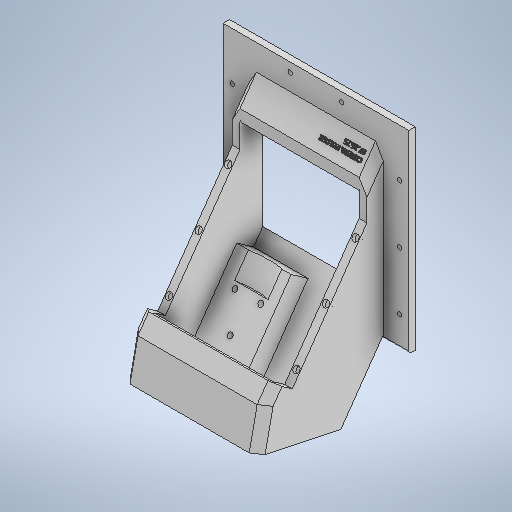
# Autodesk Inventor part: holderforcameras
Saved by Autodesk Inventor 2025.2 (Build 292293000, 293)
## iProperties
Created: 2025-07-10
Part Number: holderforcameras
Material: Generic
Document SubType Name: Modeling
Designer: mateo
Density: 1 g/cm^3
Appearance: Default
Author: mateo
Autodesk Inventor part; units mm, degrees
(part 1 of 2)
ref_plane "YZ Plane" through (0, 0, 0) normal (1, 0, 0) x (0, 1, 0)
ref_plane "XZ Plane" through (0, 0, 0) normal (0, 1, 0) x (-1, 0, 0)
ref_plane "XY Plane" through (0, 0, 0) normal (0, 0, 1) x (1, 0, 0)
sketch "Sketch1" plane through (0, 0, 0) normal (0, 0, 1) x (1, 0, 0)
  line L0 (40, -60) -> (-40, -60)
  line L1 (50, 50) -> (50, -50)
  line L2 (-50, -50) -> (-50, 50)
  line L3 (-40, 60) -> (40, 60)
  line L4 (50, -60) -> (50, 60)
  line L5 (50, 60) -> (-50, 60)
  line L6 (-50, 60) -> (-50, -60)
  line L7 (50, -60) -> (-50, -60)
  line L8 (-72, 82) -> (72, 82)
  line L9 (72, 82) -> (72, 0)
  line L10 (72, 0) -> (72, -82)
  line L11 (72, -82) -> (-72, -82)
  line L12 (-72, -82) -> (-72, 82)
  point P0 (0, 0)
  point P1 (0, 10)
  point P2 (0, 0)
  constraints: 26 end point, 3 perpendicular, 2 point on line, 1 collinear
extrude "Extrusion1" add sketch "Sketch1" along normal blind 5
sketch "Sketch2" plane through (0, 305, 5) normal (0, 0, 1) x (1, 0, 0)
  point P0 (0, 0)
  point P1 (-65, -305)
  point P2 (-65, -260)
  point P3 (-65, -350)
  point P4 (65, -305)
  point P5 (65, -260)
  point P6 (65, -350)
  point P7 (-20, -230)
  point P8 (20, -230)
  point P9 (-20, -380)
  point P10 (20, -380)
  dimension "d7" = 45
  dimension "d8" = 45
  dimension "d6" = 45
  dimension "d5" = 45
  measures "d7" distance of point (-65, -350) point (-65, -305)
  measures "d8" distance of point (-65, -305) point (-65, -260)
  measures "d6" distance of point (65, -305) point (65, -260)
  measures "d5" distance of point (65, -350) point (65, -305)
hole "Hole1" at (-65, 0, 5) at (-65, 45, 5) at (-65, -45, 5) at (65, 0, 5) at (65, 45, 5) at (65, -45, 5) at (-20, 75, 5) at (20, 75, 5) at (-20, -75, 5) at (20, -75, 5) direction (0, 0, -1) diameter 3.4587 depth 10.8 tip angle 118
move or copy body "Move Body1" bodies to move or copy 1 copy no translate (-2.5, -1.5, 0)
ref_plane "Work Plane1" through (-52.5, 58.5, 5) normal (0, -0.6427876, 0.7660444) x (1, 0, 0)
ref_plane "Work Plane2" through (47.5, -61.5, 5) normal (0, 0.5735764, 0.819152) x (-1, 0, 0)
sketch "Sketch6" plane through (47.5, -61.5, 5) normal (0, 0.5735764, 0.819152) x (-1, 0, 0)
  line L0 (102.232, 1.5875) -> (102.232, -110.9125)
  line L1 (-2.232, -110.9125) -> (-2.232, 1.5875)
  line L2 (-2.232, -110.9125) -> (102.232, -110.9125)
  line L3 (102.232, 1.5875) -> (102.232, 46.5875)
  line L4 (102.232, 46.5875) -> (-2.232, 46.5875)
  line L5 (-2.232, 46.5875) -> (-2.232, 1.5875)
  ellipse E0 centre (115, -12.2873) end of major axis (113.2706, -12.2873) minor radius 1.4166 projected
  ellipse E1 centre (-15, -12.2873) end of major axis (-16.7294, -12.2873) minor radius 1.4166 projected
  ellipse E2 centre (115, -49.1491) end of major axis (113.2706, -49.1491) minor radius 1.4166 projected
  ellipse E3 centre (-15, -49.1491) end of major axis (-16.7294, -49.1491) minor radius 1.4166 projected
  line L6 (102.232, 1.5875) -> (102.232, 46.5875)
  point P0 (47.5, -53.2457)
  dimension "d76" = 12.768
  dimension "d77" = 12.768
  dimension "d78" = 12.768
  dimension "d79" = 12.768
  constraints: 14 end point, 2 parallel, 2 perpendicular, 4 other
  measures "d76" distance from line of point (115, -12.287) L0
  measures "d77" distance from line of point (-15, -12.287) L1
  measures "d78" distance from line of L0 point (115, -49.149)
  measures "d79" distance from line of point (-15, -49.149) L1
extrude "Extrusion4" add sketch "Sketch6" along normal blind 70 contours L0 L2 L1 L5 L4 L3
sketch "Sketch8" plane through (47.5, -61.5, 5) normal (0, 0.5735764, 0.819152) x (-1, 0, 0)
  line L0 (0, -115.8875) -> (100, -115.8875) projected
  line L1 (0, -101.1661) -> (0, -2.8679) projected
  line L2 (96.232, -115.8875) -> (3.768, -115.8875)
  line L3 (102.232, 46.5875) -> (-2.232, 46.5875) projected
  line L4 (0, 46.5875) -> (100, 46.5875)
  line L5 (102.232, -110.9125) -> (102.232, -8.7172) projected
  line L6 (-2.232, -8.7172) -> (-2.232, -110.9125) projected
  line L7 (102.232, 0) -> (102.232, 46.5875) projected
  line L8 (96.232, 46.5875) -> (3.768, 46.5875)
  line L9 (3.768, 46.5875) -> (3.768, -115.8875)
  line L10 (3.768, -115.8875) -> (96.232, -115.8875)
  line L11 (96.232, -115.8875) -> (96.232, 46.5875)
  point P0 (47.5, -53.2457)
  point P1 (0, -8.7172)
  point P2 (96.232, -115.8875)
  point P3 (96.232, 46.5875)
  point P4 (3.768, 46.5875)
  point P5 (3.768, -115.8875)
  dimension "d42" = 6
  dimension "d43" = 6
  constraints: 12 end point, 2 horizontal, 2 parallel, 2 point on line, 1 perpendicular
  measures "d42" distance between parallel lines of L11 L5
  measures "d43" distance between parallel lines of L9 L6
extrude "Extrusion6" cut sketch "Sketch8" along normal blind 65
sketch "Sketch12" plane through (-54.732, -54.3593, 0) normal (-1, 0, 0) x (0, 0, 1)
  line L0 (0, 0) -> (0, 122.0413) projected
  line L1 (-1.2762, 123.8638) -> (0, 122.0413) projected
  line L2 (0, 122.0413) -> (-1.2762, 123.8638)
  line L3 (-1.2762, 123.8638) -> (-58.6698, 83.6763)
  line L4 (-58.6698, 83.6763) -> (0, -0.1129)
  line L5 (0, -0.1129) -> (0, 122.0413)
  point P0 (0, 54.3593)
  point P1 (0, 0)
  constraints: 8 end point, 2 perpendicular, 1 collinear, 1 vertical
extrude "Extrusion8" cut sketch "Sketch12" against normal through all
chamfer "Chamfer1" distance 6 angle 45 2 edges at (49.732, 0.5147, 47.0311) (-54.732, 0.5147, 47.0311)
sketch "Sketch15" plane through (47.5, -61.5, 5) normal (0, 0.5735764, 0.819152) x (-1, 0, 0)
  line L0 (96.232, -110.9125) -> (96.232, 46.5875) projected
  line L1 (3.768, -23.8125) -> (96.232, -23.8125)
  line L2 (96.232, -23.8125) -> (96.232, 11.2719)
  line L3 (3.768, 46.5875) -> (3.768, -110.9125) projected
  line L4 (3.768, 20.6375) -> (3.768, 46.5875)
  line L5 (3.768, 46.5875) -> (96.232, 46.5875)
  line L6 (96.232, 46.5875) -> (96.232, 11.2719)
  line L7 (102.232, 0) -> (102.232, 46.5875) projected
  line L8 (3.768, 46.5875) -> (3.768, -23.8125)
  point P0 (47.5, -53.2457)
  point P1 (96.6, -101.5469)
  point P2 (96.232, 46.5875)
  point P3 (2.1357, -101.5469)
  point P4 (3.768, -110.9125)
  point P5 (96.6, -100.9795)
  point P6 (2.1357, -100.9795)
  constraints: 12 end point, 1 parallel, 4 other
extrude "Extrusion11" add sketch "Sketch15" along normal blind 5 and the other way blind 3
ref_plane "Work Plane3" through (-54.732, -59.5119, 89.0621) normal (0, 0.819152, -0.5735764) x (1, 0, 0)
sketch "Sketch17" plane through (-54.732, -59.5119, 89.0621) normal (0, 0.819152, -0.5735764) x (1, 0, 0)
  line L0 (0, 70) -> (0, 6) projected
  line L1 (0, 6) -> (6, 0) projected
  line L2 (0, 6) -> (6, 0)
  line L3 (6, 0) -> (98.464, 0) projected
  line L4 (6, 0) -> (98.464, 0)
  line L5 (98.464, 0) -> (104.464, 6)
  line L6 (104.464, 6) -> (104.464, 34.8957)
  line L7 (104.464, 34.8957) -> (99.464, 34.8957)
  line L8 (6, 65) -> (6, 5) projected
  line L9 (0, 70) -> (0, 6) projected
  line L10 (0, 34.8957) -> (0, 6)
  line L11 (6, 5) -> (98.464, 5) projected
  line L12 (6, 5) -> (99.3003, 5)
  line L13 (98.464, 5) -> (98.464, 65) projected
  line L14 (6, 5) -> (6, 35)
  ellipse E0 centre (52.2321, 35) end of major axis (99.4643, 35) minor radius 30 (99.464, 34.8957) -> (99.464, 34.8957) ccw
  line L15 (99.464, 34.8957) -> (98.464, 34.8945)
  line L16 (98.464, 34.8945) -> (98.464, 5)
  line L17 (6, 5) -> (6, 35)
  line L18 (0, 34.8957) -> (6, 35)
  ellipse E1 centre (52.2319, 34.8945) end of major axis (5.9997, 34.8945) minor radius 30 (6, 35) -> (48.3586, 5) ccw
  ellipse E2 centre (52.2319, 34.8945) end of major axis (5.9997, 34.8945) minor radius 30 (56.1052, 5) -> (98.464, 34.8945) ccw
  point P0 (54.732, 38.8208)
  point P1 (5, 35)
  point P2 (5, 65)
  point P3 (0, 34.8957)
  point P4 (0, 34.8957)
  point P5 (6, 34.7891)
  point P6 (48.3586, 5)
  constraints: 24 end point, 4 perpendicular, 3 collinear, 3 point on line, 2 vertical, 16 other
extrude "Extrusion13" add sketch "Sketch17" against normal blind 15 contours L18 E0 L8 L11 L13 L7 L6 L5 L3 L1 L0 | L18 L8 E0 | L15 E0 L13 picked at (5.8412, 31.4681) picked at (98.6075, 31.369)
ref_plane "Work Plane4" through (-54.732, -99.6622, 31.7215) normal (0, -0.819152, 0.5735764) x (1, 0, 0)
ref_plane "Work Plane6" through (-54.732, -99.6622, 31.7215) normal (0, -0.9786416, 0.205574) x (1, 0, 0)
sketch "Sketch27" plane through (-54.732, -99.6622, 31.7215) normal (0, -0.9786416, 0.205574) x (1, 0, 0)
  line L0 (0, 38.1748) -> (5, 38.0788) projected
  line L1 (5, 38.0788) -> (0, 38.1748)
  line L2 (0, 4.6325) -> (0, 64.7463) projected
  line L3 (0, 38.1748) -> (0, 64.7463)
  line L4 (6, 70.2637) -> (0, 64.7463) projected
  line L5 (0, 64.7463) -> (6, 70.2637)
  line L6 (6, 70.2637) -> (98.425, 70.2637)
  line L7 (104.464, 64.7463) -> (104.464, 4.6325) projected
  line L8 (98.425, 70.2637) -> (104.464, 64.7463)
  line L9 (104.464, 64.7463) -> (104.464, 38.1748)
  line L10 (99.464, 38.1748) -> (104.464, 38.1748) projected
  line L11 (104.464, 38.1748) -> (99.464, 38.1748)
  line L12 (6, 1.5656) -> (6, 65.6659) projected
  ellipse E0 centre (52.2125, 38.1748) end of major axis (98.4632, 38.1748) minor radius 27.5938 (47.2131, 65.6069) -> (6, 39.2954) ccw
  line L13 (99.464, 38.1748) -> (99.4629, 38.3666)
  line L14 (99.4629, 38.3666) -> (99.464, 38.1748)
  line L15 (6, 65.6659) -> (98.464, 65.6659) projected
  line L16 (6, 65.6659) -> (57.4378, 65.5923)
  line L17 (99.3003, 65.6659) -> (6, 65.6659)
  line L18 (99.3003, 65.6659) -> (98.464, 65.6659)
  line L19 (98.464, 65.6659) -> (98.464, 38.1758) projected
  line L20 (99.464, 32.2809) -> (99.464, 38.1748) projected
  line L21 (5, 38.0788) -> (6, 38.0788) projected
  line L22 (5, 38.0788) -> (6, 38.0788)
  line L23 (6, 38.0788) -> (6, 65.6659)
  line L24 (98.464, 38.1758) -> (99.464, 38.1748) projected
  line L25 (98.464, 38.1758) -> (99.464, 38.1748)
  line L26 (99.464, 38.1748) -> (98.464, 38.1758)
  point P0 (54.732, -10.556)
  point P1 (48.3586, 65.6659)
  point P2 (56.1052, 65.6659)
  dimension "d91" = 5
  constraints: 32 end point, 7 collinear, 3 horizontal, 2 point on line, 1 perpendicular, 1 vertical, 7 other
  measures "d91" horizontal distance of L0.start L0.end
extrude "Extrusion21" add sketch "Sketch27" along normal mid plane 30 contours L2 L4 L6 L8 L7 L10 L24 L19 L15 L12 L21 L0
sketch "Sketch28" plane through (-54.732, -84.9826, 28.6379) normal (0, 0.9786416, -0.205574) x (1, 0, 0)
  line L0 (104.464, -64.7463) -> (104.464, -63.1884) projected
  line L1 (104.464, -64.7463) -> (104.464, -63.1884)
  line L2 (98.464, -6.7829) -> (98.464, -69.7132) projected
  line L3 (104.464, -63.1884) -> (98.464, -69.7132)
  line L4 (6, -6.7829) -> (6, -69.7132) projected
  line L5 (98.464, -69.7132) -> (6, -69.7132)
  line L6 (0, -63.1884) -> (6, -69.7132) projected
  line L7 (6, -69.7132) -> (0, -63.1884)
  line L8 (0, -63.1884) -> (0, -64.7463)
  line L9 (0, -64.7463) -> (6, -70.2637)
  line L10 (6, -70.2637) -> (98.464, -70.2637)
  line L11 (98.464, -70.2637) -> (104.464, -64.7463)
  point P0 (54.732, 10.556)
  constraints: 16 end point, 3 equal length, 3 perpendicular, 1 vertical
extrude "Extrusion22" cut sketch "Sketch28" against normal through all
sketch "Sketch31" plane through (-54.732, -61.5, 5) normal (-1, 0, 0) x (0, 0, 1)
  line L0 (26.7215, -38.1622) -> (55.4773, -18.0272) projected
  line L1 (64.0809, -30.3145) -> (67.1645, -44.9941) projected
  line L2 (26.7215, -38.1622) -> (67.1645, -44.9941)
  line L3 (55.4773, -18.0272) -> (64.0809, -30.3145) projected
  line L4 (67.0706, -45.0138) -> (94.0685, -39.3427) projected
  line L5 (70.081, -44.3815) -> (67.0706, -45.0138)
  line L6 (70.081, -44.3815) -> (63.7303, -15.5115)
  line L7 (63.7303, -15.5115) -> (25.4, -18.0272)
  line L8 (25.4, -18.0272) -> (26.7215, -38.1622)
  point P0 (-5, 61.5)
  point P1 (79.1472, -1.4534)
  constraints: 10 end point, 1 collinear, 1 perpendicular, 1 point on line
extrude "Extrusion25" add sketch "Sketch31" against normal blind 6
sketch "Sketch32" plane through (49.732, -61.5, 5) normal (1, 0, 0) x (0, 0, -1)
  line L0 (-26.7215, -38.1622) -> (0, 0) projected
  line L1 (-26.7215, -38.1622) -> (-67.1645, -44.9941) projected
  line L2 (-26.7215, -38.1622) -> (-67.1645, -44.9941)
  line L3 (-64.0809, -30.3145) -> (-67.1645, -44.9941) projected
  line L4 (-67.1645, -44.9941) -> (-64.0809, -30.3145)
  line L5 (-55.4773, -18.0272) -> (-64.0809, -30.3145) projected
  line L6 (-64.0809, -30.3145) -> (-55.4773, -18.0272)
  line L7 (-55.4773, -18.0272) -> (-26.7215, -38.1622)
  line L8 (-67.1645, -44.9941) -> (-71.4375, -44.0965)
  line L9 (-94.0685, -39.3427) -> (-67.1656, -44.9939) projected
  line L10 (-71.4375, -44.0965) -> (-64.617, -11.6275)
  line L11 (-64.617, -11.6275) -> (-26.7215, -38.1622)
  point P0 (5, 61.5)
  constraints: 14 end point, 3 collinear, 3 perpendicular, 2 point on line
extrude "Extrusion26" add sketch "Sketch32" against normal blind 6
sketch "Sketch34" plane through (47.5, -58.6321, 9.0958) normal (0, 0.5735764, 0.819152) x (1, 0, 0)
  line L0 (-3.768, 15.858) -> (-3.768, -46.5875) projected
  line L1 (-96.232, -46.5875) -> (-96.232, 15.858) projected
  line L2 (-96.232, -46.5875) -> (-3.768, -46.5875) projected
  line L3 (-3.768, 23.8125) -> (-96.232, 23.8125) projected
  line L4 (-50, -46.5875) -> (-50, 23.8125)
  line L5 (-94, -46.5875) -> (-54, -46.5875)
  line L6 (-54, -46.5875) -> (-54, 3.4125)
  line L7 (-54, 3.4125) -> (-94, 3.4125)
  line L8 (-94, 3.4125) -> (-96.232, 3.4125)
  line L9 (-96.232, 3.4125) -> (-96.232, -46.5875)
  line L10 (-94, -46.5875) -> (-96.232, -46.5875)
  point P0 (-47.5, 53.2457)
  point P1 (-54, -46.5875)
  dimension "d100" = 92.464
  dimension "d101" = 70.4
  dimension "d112" = 50
  constraints: 14 end point, 4 perpendicular, 2 midpoint, 2 point on line, 1 horizontal, 1 parallel
  measures "d100" distance between parallel lines of L0 L1
  measures "d101" distance between parallel lines of L2 L3
  measures "d112" distance between parallel lines of L2 L7
extrude "Extrusion27" add sketch "Sketch34" along normal blind 16
sketch "Sketch35" plane through (47.5, -49.4549, 22.2022) normal (0, 0.5735764, 0.819152) x (1, 0, 0)
  circle A0 centre (-74.6125, -42.8625) radius 2
  circle A1 centre (-84.6125, -19.1625) radius 2
  line L0 (-74.6125, 141.2434) -> (-74.6125, 78.7138)
  circle A2 centre (-64.6125, -19.1625) radius 2
  line L1 (-220.5298, -133.1321) -> (71.3048, -56.0245)
  point P0 (-47.5, 53.2457)
  point P1 (-90.1769, -210.863)
  point P2 (-74.6125, -94.5783)
  point P3 (-74.6125, -94.5783)
  dimension "d115" = 4
  dimension "d117" = 4
  dimension "d121" = 50
  dimension "d122" = 20
  dimension "d123" = 23.7
  constraints: 4 end point, 3 centre point, 2 midpoint, 2 vertical alignment, 1 symmetric about line, 1 vertical, 1 other
  measures "d115" diameter of A0
  measures "d117" diameter of A1
  measures "d121" distance from line of L1 A0.centre
  measures "d122" distance of A2.centre A1.centre
  measures "d123" vertical distance of A0.centre A1.centre
extrude "Extrusion28" cut sketch "Sketch35" against normal blind 24.6695
sketch "Sketch36" plane through (-74.5, -83.5, 5) normal (0, 0, 1) x (1, 0, 0)
  line L0 (22, 22) -> (19.768, 22) projected
  line L1 (124.232, 0) -> (19.768, 0)
  line L2 (124.232, 13.701) -> (19.768, 13.701)
  line L3 (19.768, 13.701) -> (0, 13.701)
  line L4 (0, 164) -> (0, 0) projected
  line L5 (0, 13.701) -> (0, 0)
  line L6 (0, 0) -> (19.768, 0)
  line L7 (0, 0) -> (144, 0) projected
  line L8 (124.232, 13.701) -> (144, 13.701)
  line L9 (144, 0) -> (144, 164) projected
  line L10 (144, 13.701) -> (144, 0)
  line L11 (144, 0) -> (124.232, 0)
  point P0 (74.5, 83.5)
  point P1 (0, 13.701)
  constraints: 16 end point, 3 collinear, 2 point on line, 1 perpendicular
sketch "Sketch37" plane through (-49.732, -99.6622, 31.7215) normal (0, -0.819152, 0.5735764) x (1, 0, 0)
  line L0 (-5, 0) -> (99.464, 0) projected
  line L1 (0, 8) -> (0, 0)
  line L2 (94.464, 0) -> (94.4704, 0)
  line L3 (-5, 0) -> (99.464, 0) projected
  line L4 (94.4704, 0) -> (94.464, 0)
  line L5 (93.464, 0) -> (93.464, 5)
  line L6 (93.464, 0) -> (93.464, 5) projected
  line L7 (93.464, 5) -> (43.232, 5)
  line L8 (43.232, 5) -> (43.232, 21)
  line L9 (43.232, 5) -> (93.464, 5) projected
  line L10 (0, 8) -> (0, 0)
  line L11 (1, 21) -> (4.232, 21)
  line L12 (1, 8) -> (1, 21)
  line L13 (1, 29.137) -> (1, 0) projected
  line L14 (1, -3) -> (1, 5) projected
  line L15 (0, 0) -> (0, -3)
  line L16 (93.464, -3) -> (93.464, 5) projected
  line L17 (1, -3) -> (93.464, -3)
  line L18 (93.464, -3) -> (93.464, 5)
  line L19 (1, 21) -> (43.232, 21)
  line L20 (-5, 0) -> (-5, 29.2104) projected
  line L21 (1, 21) -> (1, -3)
  line L22 (93.464, -3) -> (93.464, 5)
  line L23 (43.232, 5) -> (43.232, 21)
  point P0 (49.732, 31.1792)
  point P1 (0, 29.137)
  point P2 (1, 5)
  point P3 (0, 8)
  point P4 (93.464, 41.1414)
  point P5 (93.464, 65)
  point P6 (1, 29.2104)
  point P7 (93.464, 35.1055)
  point P8 (1, 0)
  point P9 (1, 0)
  point P10 (93.464, 0)
  constraints: 30 end point, 4 vertical, 3 collinear, 3 horizontal, 3 perpendicular, 1 point on line, 10 other
extrude "Extrusion29" add sketch "Sketch37" along normal blind 15
sketch "Sketch38" plane through (-49.732, -111.9495, 40.3251) normal (0, -0.819152, 0.5735764) x (1, 0, 0)
  line L0 (3.232, 8) -> (3.232, 24) projected
  line L1 (43.232, 5) -> (43.232, 21) projected
  line L2 (3.232, 24) -> (43.232, 24)
  line L3 (43.232, 24) -> (43.232, 22.05)
  line L4 (43.232, 22.05) -> (3.232, 22.05)
  line L5 (3.232, 22.05) -> (3.232, 24)
  point P0 (49.732, 31.1792)
  point P1 (3.232, 22.05)
  dimension "d141" = 16
  constraints: 8 end point, 2 parallel, 1 horizontal, 1 perpendicular, 1 point on line
  measures "d141" distance of L0.start L0.end
extrude "Extrusion30" cut sketch "Sketch38" against normal blind 288.2125
extrude "Extrusion31" cut sketch "Sketch36" against normal blind 288.2125
sketch "Sketch40" plane through (47.5, -61.5, 5) normal (0, -0.5735764, -0.819152) x (-1, 0, 0)
  circle A0 centre (74.6125, -42.8625) radius 2 projected
  circle A1 centre (64.6125, -19.1625) radius 2 projected
  circle A2 centre (84.6125, -19.1625) radius 2 projected
  circle A3 centre (74.6125, -42.8625) radius 5.5
  circle A4 centre (84.6125, -19.1625) radius 5.5
  circle A5 centre (64.6125, -19.1625) radius 5.5
  point P0 (47.5, 53.2457)
  dimension "d136" = 11
  dimension "d137" = 11
  dimension "d138" = 11
  constraints: 3 centre point, 3 coincident
  measures "d136" diameter of A3
  measures "d137" diameter of A4
  measures "d138" diameter of A5
extrude "Extrusion32" cut sketch "Sketch40" along normal blind 10 and the other way blind 5
fillet "Fillet1" radius 2 1 edges at (-2.5, -69.799, 5)
sketch "Sketch41" plane through (47.5, -58.6321, 9.0958) normal (0, 0.5735764, 0.819152) x (1, 0, 0)
  line L0 (-54, 3.4125) -> (-54, -61.5875) projected
  line L1 (22, -5.1598) -> (-122, -5.1598) projected
  line L2 (-3.768, -61.5875) -> (-54, -61.5875) projected
  circle A0 centre (-29.5, -43.75) radius 3.5
  circle A1 centre (-29.5, -15.75) radius 3.5
  point P0 (-47.5, 53.2457)
  dimension "d147" = 7
  dimension "d149" = 7
  dimension "d196" = 28
  constraints: 2 centre point
  measures "d147" diameter of A0
  measures "d149" diameter of A1
  measures "d196" distance of A1.centre A0.centre
extrude "Extrusion33" cut sketch "Sketch41" against normal through all
sketch "Sketch42" plane through (47.5, -61.5, 5) normal (0, -0.5735764, -0.819152) x (-1, 0, 0)
  line L0 (97.232, -46.5875) -> (2.768, -46.5875) projected
  arc A0 (33, -43.75) -> (33, -43.75) centre (29.5, -43.75) ccw projected
  arc A1 (26, -43.75) -> (26, -43.75) centre (29.5, -43.75) ccw projected
  circle A2 centre (29.5, -43.75) radius 7.5
  circle A3 centre (29.5, -15.75) radius 3.5 projected
  circle A4 centre (29.5, -15.75) radius 7.5
  point P0 (47.5, 53.2457)
  point P1 (2.768, -46.5875)
  dimension "d158" = 15
  dimension "d197" = 15
  constraints: 2 centre point, 2 coincident, 1 other
  measures "d158" diameter of A2
  measures "d197" diameter of A4
extrude "Extrusion34" cut sketch "Sketch42" along normal blind 5 and the other way blind 3
sketch "Sketch44" plane through (47.5, -61.5, 5) normal (0, -0.5735764, -0.819152) x (-1, 0, 0)
  line L0 (102.232, -46.5875) -> (96.232, -46.5875) projected
  line L1 (96.232, 0) -> (96.232, -46.5875) projected
  line L2 (102.232, 0) -> (102.232, -46.5875) projected
  line L3 (100, 0) -> (102.232, 0) projected
  line L4 (96.232, 0) -> (100, 0) projected
  line L5 (100, 8.7172) -> (96.232, 8.7172) projected
  line L6 (96.232, 8.7172) -> (96.232, 0) projected
  line L7 (100, 8.7172) -> (100, 0) projected
  line L8 (96.232, 0) -> (96.232, 2.1006) projected
  line L9 (102.232, -46.5875) -> (96.232, -46.5875)
  line L10 (96.232, -46.5875) -> (96.232, 0)
  line L11 (96.232, 0) -> (102.232, 0)
  line L12 (102.232, 0) -> (102.232, -46.5875)
  line L13 (3.768, -46.5875) -> (3.768, 0) projected
  line L14 (0, 0) -> (3.768, 0) projected
  line L15 (-2.232, 0) -> (0, 0) projected
  line L16 (-2.232, -46.5875) -> (-2.232, 0) projected
  line L17 (3.768, 8.7172) -> (0, 8.7172) projected
  line L18 (0, 0) -> (0, 8.7172) projected
  line L19 (3.768, 0) -> (3.768, 8.7172) projected
  line L20 (2.768, -46.5875) -> (-2.232, -46.5875)
  line L21 (-2.232, -46.5875) -> (-2.232, 0)
  line L22 (-2.232, 0) -> (2.768, 0)
  line L23 (2.768, 0) -> (2.768, -46.5875)
  line L24 (96.232, 0) -> (100, 0) projected
  line L25 (102.232, -46.5875) -> (96.232, -46.5875)
  line L26 (96.232, -46.5875) -> (96.232, 0)
  line L27 (96.232, 0) -> (102.232, 0)
  line L28 (102.232, 0) -> (102.232, -46.5875)
  line L29 (-2.232, -46.5875) -> (-2.232, 0) projected
  line L30 (2.768, -46.5875) -> (-2.232, -46.5875)
  line L31 (-2.232, -46.5875) -> (-2.232, 0)
  line L32 (-2.232, 0) -> (2.768, 0)
  line L33 (2.768, 0) -> (2.768, -46.5875)
  line L34 (96.232, 0) -> (96.232, -46.5875) projected
  line L35 (102.232, 0) -> (102.232, -46.5875) projected
  line L36 (100, 0) -> (102.232, 0) projected
  line L37 (96.232, 0) -> (100, 0) projected
  line L38 (102.232, -46.5875) -> (96.232, -46.5875) projected
  line L39 (3.768, -46.5875) -> (-2.232, -46.5875) projected
  line L40 (100, 8.7172) -> (96.232, 8.7172) projected
  line L41 (96.232, 8.7172) -> (96.232, 0) projected
  line L42 (100, 8.7172) -> (100, 0) projected
  line L43 (3.768, -46.5875) -> (3.768, 0) projected
  line L44 (0, 0) -> (3.768, 0) projected
  line L45 (-2.232, 0) -> (0, 0) projected
  line L46 (-2.232, -46.5875) -> (-2.232, 0) projected
  line L47 (102.232, -46.5875) -> (96.232, -46.5875) projected
  line L48 (3.768, -46.5875) -> (-2.232, -46.5875) projected
  line L49 (3.768, 8.7172) -> (0, 8.7172) projected
  line L50 (0, 0) -> (0, 8.7172) projected
  line L51 (3.768, 0) -> (3.768, 8.7172) projected
  point P0 (47.5, 53.2457)
  point P1 (102.232, -46.5875)
  point P2 (2.768, 0)
  constraints: 32 end point, 8 parallel, 4 horizontal, 4 perpendicular
extrude "Extrusion35" add sketch "Sketch44" along normal blind 3 contours L0 L1 L4 L3 L2 | L39 L23 L14 L13 | L20 L16 L15 L14 L23
sketch "Sketch45" plane through (44.732, -106.4941, 72.1645) normal (0, -0.9860303, -0.166566) x (1, 0, 0)
  line L0 (-99.464, -41.016) -> (-99.464, 0) projected
  line L1 (-99.464, -41.016) -> (5, -41.016) projected
  line L2 (5, 0) -> (5, -41.016) projected
  line L3 (-1, -33.9952) -> (-1, 0) projected
  line L4 (-1, -41.016) -> (5, -41.016) projected
  line L5 (-99.464, 0) -> (-93.464, 0)
  line L6 (-99.464, -41.016) -> (-99.464, 0)
  line L7 (5, 0) -> (5, -41.016) projected
  line L8 (0, 0) -> (5, 0)
  line L9 (5, 0) -> (5, -41.016)
  line L10 (-1, 0) -> (5, 0) projected
  line L11 (-1, -41.016) -> (-1, -33.9952) projected
  line L12 (5, -72.8496) -> (5, -43.1525) projected
  line L13 (5, -43.1525) -> (-99.464, -43.1525) projected
  line L14 (5, -43.1525) -> (-1, -43.1525)
  line L15 (-1, -43.1525) -> (-1, 0)
  line L16 (5, 0) -> (5, -43.1525)
  line L17 (5, -43.1525) -> (-99.464, -43.1525) projected
  line L18 (-99.464, -41.016) -> (-99.464, -43.1525)
  line L19 (-99.464, -43.1525) -> (-93.464, -43.1525)
  line L20 (-93.464, -43.1525) -> (-93.464, -41.016)
  line L21 (-93.464, 0) -> (-99.464, 0)
  line L22 (-99.464, 0) -> (-99.464, -43.1525)
  line L23 (-99.464, -43.1525) -> (-93.464, -43.1525)
  line L24 (-93.464, 0) -> (-93.464, -43.1525)
  line L25 (-93.464, -98.7163) -> (-93.464, 15.8051) projected
  point P0 (-44.732, -88.8947)
  point P1 (-94.464, -0.1031)
  point P2 (-94.464, -41.016)
  point P3 (-93.464, -0.1031)
  point P4 (5, -41.016)
  point P5 (-1, -41.016)
  point P6 (-93.464, -41.016)
  point P7 (-99.464, -41.016)
  constraints: 28 end point, 7 collinear, 3 horizontal, 1 perpendicular, 1 vertical
extrude "Extrusion37" add sketch "Sketch45" along normal blind 15 contours L0 L5 L24 L1 | L1 L20 L13 L18 | L11 L3 L10 L8 L2 L1 | L1 L16 L13 L15
sketch "Sketch47" plane through (49.732, -66.7303, 5) normal (1, 0, 0) x (0, 0, -1)
  line L0 (-67.0629, -39.7466) -> (-67.0706, -39.7835) projected
  line L1 (-67.0706, -39.7835) -> (-27.0245, -48.1956)
  line L2 (-64.6661, -54.5542) -> (-22.1163, -47.3665) projected
  line L3 (-27.0245, -48.1956) -> (-64.578, -54.5394)
  line L4 (-67.1645, -39.7638) -> (-94.0685, -34.1123) projected
  line L5 (-64.578, -54.5394) -> (-64.6661, -54.5542)
  line L6 (-67.1645, -39.7638) -> (-64.6661, -54.5542) projected
  line L7 (-67.1645, -39.7638) -> (-67.0706, -39.7835)
  point P0 (5, 66.7303)
  point P1 (-32.8677, -46.9399)
  point P2 (-24.223, -47.7224)
  point P3 (-63.9955, -25.144)
  constraints: 8 end point, 2 collinear, 1 point on line
extrude "Extrusion38" cut sketch "Sketch47" against normal blind 120
sketch "Sketch49" plane through (-48.732, -54.3593, 0) normal (-1, 0, 0) x (0, 0, 1)
  line L0 (0, 8.7172) -> (44.4209, -54.7224) projected
  line L1 (0, 8.7172) -> (0, -5.2303)
  line L2 (1.3377, -7.1407) -> (-11.1157, 10.6446) projected
  line L3 (-11.1157, 10.6446) -> (-4.3813, 15.3601)
  line L4 (-4.3813, 15.3601) -> (0, 8.7172)
  line L5 (0, 8.7172) -> (-4.5625, 15.2332) projected
  line L6 (-11.1157, 10.6446) -> (0, -5.2303)
  point P0 (0, 54.3593)
  constraints: 8 end point, 3 point on line, 2 perpendicular, 1 vertical
extrude "Extrusion40" cut sketch "Sketch49" against normal through all contours L1 L2 L3 L5
sketch "Sketch50" plane through (-48.732, -55.8368, 7.1384) normal (0, 0.819152, -0.5735764) x (1, 0, 0)
  line L0 (42.232, -16) -> (0, -16) projected
  line L1 (9.0575, -16) -> (7.9375, -16)
  arc A0 (34.925, -16) -> (9.0575, -16) centre (21.9913, -30.5193) ccw
  line L2 (34.925, -16) -> (9.0575, -16)
  point P0 (48.732, -26.1792)
  point P1 (33.6195, -16)
  point P2 (9.0575, -16)
  constraints: 4 end point, 2 point on circle, 2 point on line, 1 centre point
extrude "Extrusion41" cut sketch "Sketch50" against normal blind 18.575
sketch "Sketch52" plane through (-54.732, -66.7303, 5) normal (-1, 0, 0) x (0, 0, 1)
  line L0 (26.7215, -32.9319) -> (24.223, -47.7224) projected
  line L1 (27.0245, -48.1956) -> (94.0685, -34.1123) projected
  line L2 (24.223, -47.7224) -> (27.0245, -48.1956) projected
  line L3 (32.8677, -46.9399) -> (26.0097, -37.1457) projected
  line L4 (26.0097, -37.1457) -> (32.8677, -46.9399)
  line L5 (27.0245, -48.1956) -> (24.223, -47.7224)
  line L6 (26.0097, -37.1457) -> (24.223, -47.7224)
  line L7 (32.8677, -46.9399) -> (32.9391, -47.042)
  line L8 (32.9391, -47.042) -> (27.0245, -48.1956)
  point P0 (-5, 66.7303)
  point P1 (32.8849, -46.9646)
  constraints: 10 end point, 2 collinear, 1 perpendicular, 1 point on line
extrude "Extrusion43" cut sketch "Sketch52" against normal through all contours L3 L7 L1 L2 L0
sketch "Sketch53" plane through (-54.732, -66.7303, 5) normal (-1, 0, 0) x (0, 0, 1)
  line L0 (0, 116.8109) -> (85.4767, -5.2624) projected
  line L1 (12.7, 98.6735) -> (85.4767, -5.2624)
  line L2 (12.7, 81.631) -> (70.555, -0.9945)
  line L3 (12.7, 81.631) -> (12.7, 130.812)
  line L4 (70.555, -0.9945) -> (93.6625, 15.1855)
  line L5 (12.7, 130.812) -> (93.6625, 15.1855)
  line L6 (70.555, -0.9945) -> (12.7, 81.631)
  line L7 (12.7, 130.812) -> (12.7, 81.631)
  point P0 (-5, 66.7303)
  point P1 (87.7509, -8.5103)
  constraints: 14 end point, 2 collinear, 2 perpendicular, 2 point on line, 1 parallel
extrude "Extrusion44" cut sketch "Sketch53" against normal through all
sketch "Sketch56" plane through (-54.732, -66.7303, 5) normal (-1, 0, 0) x (0, 0, 1)
  line L0 (24.264, -34.6526) -> (22.1163, -47.3665) projected
  line L1 (24.223, -47.7224) -> (26.0097, -37.1457) projected
  line L2 (24.264, -34.6526) -> (26.0097, -37.1457)
  line L3 (26.0097, -37.1457) -> (24.223, -47.7224)
  line L4 (24.223, -47.7224) -> (21.9676, -47.3414)
  line L5 (21.9676, -47.3414) -> (24.264, -34.6526)
  point P0 (-5, 66.7303)
  constraints: 8 end point, 1 collinear, 1 perpendicular
extrude "Extrusion46" cut sketch "Sketch56" against normal through all contours L2 L1 L4 L0
sketch "Sketch57" plane through (43.732, -67.7248, 75.555) normal (0, 0.5735764, 0.819152) x (1, 0, 0)
  line L0 (6, 100.8671) -> (6, 0) projected
  line L1 (3.175, 90.4335) -> (3.175, 70.4335) construction
  line L2 (3.175, 70.4335) -> (3.175, 50.4335) construction
  line L3 (3.175, 50.4335) -> (3.175, 30.4335) construction
  line L4 (3.175, 30.4335) -> (3.175, 50.4335) construction
  line L5 (3.175, 30.4335) -> (3.175, 10.4335) construction
  line L6 (6, 0) -> (0, 0) construction
  line L7 (0, 100.8671) -> (6, 100.8671) construction
  circle A0 centre (3.175, 90.4335) radius 2.5
  circle A1 centre (3.175, 70.4335) radius 2.5
  circle A2 centre (3.175, 50.4335) radius 2.5
  circle A3 centre (3.175, 30.4335) radius 2.5
  circle A4 centre (3.175, 10.4335) radius 2.5
  line L8 (-98.464, 0) -> (-98.464, 100.8671) projected
  line L9 (6, 61.4258) -> (3.175, 61.4258)
  line L10 (0, 61.4258) -> (-92.464, 61.4258) projected
  line L11 (-50.232, 48.9803) -> (-50.232, -16.0197) projected
  circle A5 centre (-95.639, 90.4335) radius 2.5
  circle A6 centre (-95.639, 70.4335) radius 2.5
  circle A7 centre (-95.639, 50.4335) radius 2.5
  circle A8 centre (-95.639, 30.4335) radius 2.5
  circle A9 centre (-95.639, 10.4335) radius 2.5
  point P0 (3, 0)
  point P1 (3, 100.8671)
  dimension "d202" = 20
  dimension "d203" = 20
  dimension "d204" = 20
  dimension "d205" = 20
  dimension "d206" = 20
  dimension "d207" = 10.4335
  dimension "d208" = 10.4336
  dimension "d209" = 5
  dimension "d210" = 5
  dimension "d211" = 5
  dimension "d212" = 5
  dimension "d213" = 5
  constraints: 12 end point, 10 centre point, 5 coincident, 4 point on line, 2 midpoint, 2 vertical, 1 collinear
  measures "d202" distance of L1.start L1.end
  measures "d203" distance of L1.end L2.end
  measures "d204" distance of L2.end L3.end
  measures "d205" distance of L3.end L2.end
  measures "d206" distance of L3.end L5.end
  measures "d207" vertical distance of L5.end point (3, 0)
  measures "d208" vertical distance of L1.start point (3, 100.867)
  measures "d209" diameter of A0
  measures "d210" diameter of A1
  measures "d211" diameter of A2
  measures "d212" diameter of A3
  measures "d213" diameter of A4
sketch "Sketch58" plane through (47.5, -21.3496, 62.3406) normal (0, 0.5735764, 0.819152) x (1, 0, 0)
  line L0 (-6.4076, 82.6491) -> (-90.4873, 82.6491) construction
  line L1 (-90.4873, 82.6491) -> (-90.4873, 95.3086) construction
  line L2 (-90.4873, 95.3086) -> (-6.4076, 95.3086) construction
  line L3 (-6.4076, 95.3086) -> (-6.4076, 82.6491) construction
  spline S0 degree 2 poles (-7.9069, 88.048) (-7.6105, 88.048) (-7.109, 87.8479) (-6.9263, 87.6478) knots 0 0 0 1 2 2 2
  spline S1 degree 2 poles (-6.9263, 87.6478) (-6.7435, 87.4502) (-6.5434, 86.8574) (-6.5434, 86.4721) knots 0 0 0 1 2 2 2
  spline S2 degree 2 poles (-6.5434, 86.4721) (-6.5434, 86.0893) (-6.7385, 85.5212) (-6.9238, 85.3112) knots 0 0 0 1 2 2 2
  spline S3 degree 2 poles (-6.9238, 85.3112) (-7.1066, 85.1062) (-7.6055, 84.8913) (-7.9143, 84.8913) knots 0 0 0 1 2 2 2
  spline S4 degree 2 poles (-7.9143, 84.8913) (-8.0674, 84.8913) (-8.3366, 84.9358) (-8.4503, 84.9703) knots 0 0 0 1 2 2 2
  spline S5 degree 2 poles (-8.4503, 84.9703) (-8.5491, 85.0025) (-8.7541, 85.0938) (-8.8554, 85.1482) knots 0 0 0 1 2 2 2
  line L4 (-8.8554, 85.1482) -> (-8.8554, 85.6373)
  line L5 (-8.8554, 85.6373) -> (-8.8232, 85.6373)
  spline S6 degree 2 poles (-8.8232, 85.6373) (-8.7689, 85.5879) (-8.6009, 85.4495) (-8.4799, 85.3828) knots 0 0 0 1 2 2 2
  spline S7 degree 2 poles (-8.4799, 85.3828) (-8.3638, 85.3186) (-8.0896, 85.2371) (-7.9118, 85.2371) knots 0 0 0 1 2 2 2
  spline S8 degree 2 poles (-7.9118, 85.2371) (-7.7167, 85.2371) (-7.3684, 85.3977) (-7.2375, 85.5508) knots 0 0 0 1 2 2 2
  spline S9 degree 2 poles (-7.2375, 85.5508) (-7.109, 85.7064) (-6.9658, 86.1782) (-6.9658, 86.4721) knots 0 0 0 1 2 2 2
  spline S10 degree 2 poles (-6.9658, 86.4721) (-6.9658, 86.7858) (-7.1165, 87.2378) (-7.2474, 87.3934) knots 0 0 0 1 2 2 2
  spline S11 degree 2 poles (-7.2474, 87.3934) (-7.3758, 87.5441) (-7.7191, 87.6972) (-7.9118, 87.6972) knots 0 0 0 1 2 2 2
  spline S12 degree 2 poles (-7.9118, 87.6972) (-8.0872, 87.6972) (-8.386, 87.6108) (-8.5021, 87.5466) knots 0 0 0 1 2 2 2
  spline S13 degree 2 poles (-8.5021, 87.5466) (-8.6133, 87.4824) (-8.7788, 87.349) (-8.8257, 87.302) knots 0 0 0 1 2 2 2
  line L6 (-8.8257, 87.302) -> (-8.8554, 87.302)
  line L7 (-8.8554, 87.302) -> (-8.8554, 87.7862)
  spline S14 degree 2 poles (-8.8554, 87.7862) (-8.7541, 87.8331) (-8.5762, 87.9195) (-8.4503, 87.9591) knots 0 0 0 1 2 2 2
  spline S15 degree 2 poles (-8.4503, 87.9591) (-8.3169, 88.0035) (-8.0896, 88.048) (-7.9069, 88.048) knots 0 0 0 1 2 2 2
  line L8 (-8.9048, 87.9936) -> (-9.9323, 84.9456)
  line L9 (-9.9323, 84.9456) -> (-10.4312, 84.9456)
  line L10 (-10.4312, 84.9456) -> (-11.4587, 87.9936)
  line L11 (-11.4587, 87.9936) -> (-11.0314, 87.9936)
  line L12 (-11.0314, 87.9936) -> (-10.7548, 87.1415)
  line L13 (-10.7548, 87.1415) -> (-9.5914, 87.1415)
  line L14 (-9.5914, 87.1415) -> (-9.3148, 87.9936)
  line L15 (-9.3148, 87.9936) -> (-8.9048, 87.9936)
  line L16 (-10.6436, 86.7957) -> (-10.1719, 85.3606)
  line L17 (-10.1719, 85.3606) -> (-9.7026, 86.7957)
  line L18 (-9.7026, 86.7957) -> (-10.6436, 86.7957)
  line L19 (-14.361, 87.9936) -> (-13.9559, 87.9936)
  line L20 (-13.9559, 87.9936) -> (-13.9559, 85.368)
  line L21 (-13.9559, 85.368) -> (-13.1606, 87.1538)
  line L22 (-13.1606, 87.1538) -> (-12.9136, 87.1538)
  line L23 (-12.9136, 87.1538) -> (-12.1257, 85.368)
  line L24 (-12.1257, 85.368) -> (-12.1257, 87.9936)
  line L25 (-12.1257, 87.9936) -> (-11.7477, 87.9936)
  line L26 (-11.7477, 87.9936) -> (-11.7477, 84.9456)
  line L27 (-11.7477, 84.9456) -> (-12.301, 84.9456)
  line L28 (-12.301, 84.9456) -> (-13.0618, 86.6425)
  line L29 (-13.0618, 86.6425) -> (-13.7979, 84.9456)
  line L30 (-13.7979, 84.9456) -> (-14.361, 84.9456)
  line L31 (-14.361, 84.9456) -> (-14.361, 87.9936)
  line L32 (-14.9785, 87.9936) -> (-14.9785, 84.9456)
  line L33 (-14.9785, 84.9456) -> (-16.8854, 84.9456)
  line L34 (-16.8854, 84.9456) -> (-16.8854, 85.3063)
  line L35 (-16.8854, 85.3063) -> (-15.3836, 85.3063)
  line L36 (-15.3836, 85.3063) -> (-15.3836, 86.1411)
  line L37 (-15.3836, 86.1411) -> (-16.7841, 86.1411)
  line L38 (-16.7841, 86.1411) -> (-16.7841, 86.5018)
  line L39 (-16.7841, 86.5018) -> (-15.3836, 86.5018)
  line L40 (-15.3836, 86.5018) -> (-15.3836, 87.633)
  line L41 (-15.3836, 87.633) -> (-16.8854, 87.633)
  line L42 (-16.8854, 87.633) -> (-16.8854, 87.9936)
  line L43 (-16.8854, 87.9936) -> (-14.9785, 87.9936)
  line L44 (-19.6888, 87.9936) -> (-19.1627, 87.9936)
  line L45 (-19.1627, 87.9936) -> (-18.1994, 86.7809)
  line L46 (-18.1994, 86.7809) -> (-17.7351, 86.7809)
  line L47 (-17.7351, 86.7809) -> (-17.7351, 87.9936)
  line L48 (-17.7351, 87.9936) -> (-17.33, 87.9936)
  line L49 (-17.33, 87.9936) -> (-17.33, 84.9456)
  line L50 (-17.33, 84.9456) -> (-18.1154, 84.9456)
  spline S16 degree 2 poles (-18.1154, 84.9456) (-18.3773, 84.9456) (-18.7305, 85.0025) (-18.891, 85.1062) knots 0 0 0 1 2 2 2
  spline S17 degree 2 poles (-18.891, 85.1062) (-19.0516, 85.2099) (-19.2368, 85.5335) (-19.2368, 85.7731) knots 0 0 0 1 2 2 2
  spline S18 degree 2 poles (-19.2368, 85.7731) (-19.2368, 86.1066) (-18.896, 86.5586) (-18.6045, 86.6672) knots 0 0 0 1 2 2 2
  line L51 (-18.6045, 86.6672) -> (-19.6888, 87.9936)
  spline S19 degree 2 poles (-18.8145, 85.8052) (-18.8145, 85.6718) (-18.7206, 85.4668) (-18.6218, 85.4001) knots 0 0 0 1 2 2 2
  spline S20 degree 2 poles (-18.6218, 85.4001) (-18.5353, 85.3433) (-18.3056, 85.2964) (-18.1377, 85.2964) knots 0 0 0 1 2 2 2
  line L52 (-18.1377, 85.2964) -> (-17.7351, 85.2964)
  line L53 (-17.7351, 85.2964) -> (-17.7351, 86.4425)
  line L54 (-17.7351, 86.4425) -> (-18.0907, 86.4425)
  spline S21 degree 2 poles (-18.0907, 86.4425) (-18.2661, 86.4425) (-18.5452, 86.3807) (-18.6416, 86.2844) knots 0 0 0 1 2 2 2
  spline S22 degree 2 poles (-18.6416, 86.2844) (-18.7305, 86.2004) (-18.8145, 85.9633) (-18.8145, 85.8052) knots 0 0 0 1 2 2 2
  line L55 (-19.6024, 87.9936) -> (-20.6299, 84.9456)
  line L56 (-20.6299, 84.9456) -> (-21.1289, 84.9456)
  line L57 (-21.1289, 84.9456) -> (-22.1564, 87.9936)
  line L58 (-22.1564, 87.9936) -> (-21.7291, 87.9936)
  line L59 (-21.7291, 87.9936) -> (-21.4524, 87.1415)
  line L60 (-21.4524, 87.1415) -> (-20.2891, 87.1415)
  line L61 (-20.2891, 87.1415) -> (-20.0124, 87.9936)
  line L62 (-20.0124, 87.9936) -> (-19.6024, 87.9936)
  line L63 (-21.3413, 86.7957) -> (-20.8695, 85.3606)
  line L64 (-20.8695, 85.3606) -> (-20.4002, 86.7957)
  line L65 (-20.4002, 86.7957) -> (-21.3413, 86.7957)
  line L66 (-25.9676, 87.9936) -> (-25.5625, 87.9936)
  line L67 (-25.5625, 87.9936) -> (-25.5625, 86.5018)
  line L68 (-25.5625, 86.5018) -> (-24.1596, 86.5018)
  line L69 (-24.1596, 86.5018) -> (-24.1596, 87.9936)
  line L70 (-24.1596, 87.9936) -> (-23.7545, 87.9936)
  line L71 (-23.7545, 87.9936) -> (-23.7545, 84.9456)
  line L72 (-23.7545, 84.9456) -> (-24.1596, 84.9456)
  line L73 (-24.1596, 84.9456) -> (-24.1596, 86.1411)
  line L74 (-24.1596, 86.1411) -> (-25.5625, 86.1411)
  line L75 (-25.5625, 86.1411) -> (-25.5625, 84.9456)
  line L76 (-25.5625, 84.9456) -> (-25.9676, 84.9456)
  line L77 (-25.9676, 84.9456) -> (-25.9676, 87.9936)
  spline S23 degree 2 poles (-28.7415, 85.2939) (-28.9144, 85.4965) (-29.107, 86.0893) (-29.107, 86.4696) knots 0 0 0 1 2 2 2
  spline S24 degree 2 poles (-29.107, 86.4696) (-29.107, 86.8401) (-28.9193, 87.4404) (-28.7415, 87.6429) knots 0 0 0 1 2 2 2
  spline S25 degree 2 poles (-28.7415, 87.6429) (-28.5537, 87.8553) (-28.0573, 88.0579) (-27.7584, 88.0579) knots 0 0 0 1 2 2 2
  spline S26 degree 2 poles (-27.7584, 88.0579) (-27.4496, 88.0579) (-26.9556, 87.8479) (-26.7753, 87.6429) knots 0 0 0 1 2 2 2
  spline S27 degree 2 poles (-26.7753, 87.6429) (-26.5999, 87.4404) (-26.4122, 86.8451) (-26.4122, 86.4696) knots 0 0 0 1 2 2 2
  spline S28 degree 2 poles (-26.4122, 86.4696) (-26.4122, 86.0868) (-26.6024, 85.5039) (-26.7778, 85.2939) knots 0 0 0 1 2 2 2
  spline S29 degree 2 poles (-26.7778, 85.2939) (-26.9556, 85.0914) (-27.4521, 84.8814) (-27.7584, 84.8814) knots 0 0 0 1 2 2 2
  spline S30 degree 2 poles (-27.7584, 84.8814) (-28.0696, 84.8814) (-28.5686, 85.0988) (-28.7415, 85.2939) knots 0 0 0 1 2 2 2
  spline S31 degree 2 poles (-28.6846, 86.4696) (-28.6846, 86.1683) (-28.5537, 85.7015) (-28.4352, 85.5483) knots 0 0 0 1 2 2 2
  spline S32 degree 2 poles (-28.4352, 85.5483) (-28.3141, 85.3902) (-27.9733, 85.2322) (-27.7609, 85.2322) knots 0 0 0 1 2 2 2
  spline S33 degree 2 poles (-27.7609, 85.2322) (-27.541, 85.2322) (-27.21, 85.3853) (-27.0841, 85.5483) knots 0 0 0 1 2 2 2
  spline S34 degree 2 poles (-27.0841, 85.5483) (-26.963, 85.7039) (-26.8346, 86.1732) (-26.8346, 86.4696) knots 0 0 0 1 2 2 2
  spline S35 degree 2 poles (-26.8346, 86.4696) (-26.8346, 87.0699) (-27.3385, 87.7071) (-27.7609, 87.7071) knots 0 0 0 1 2 2 2
  spline S36 degree 2 poles (-27.7609, 87.7071) (-28.1832, 87.7071) (-28.6846, 87.0699) (-28.6846, 86.4696) knots 0 0 0 1 2 2 2
  line L78 (-31.3177, 87.9936) -> (-29.5516, 87.9936)
  line L79 (-29.5516, 87.9936) -> (-29.5516, 84.9456)
  line L80 (-29.5516, 84.9456) -> (-29.9567, 84.9456)
  line L81 (-29.9567, 84.9456) -> (-29.9567, 87.633)
  line L82 (-29.9567, 87.633) -> (-31.3177, 87.633)
  line L83 (-31.3177, 87.633) -> (-31.3177, 87.9936)
  spline S37 degree 2 poles (-34.0396, 86.4721) (-34.0396, 86.8895) (-33.7012, 87.5614) (-33.4172, 87.7491) knots 0 0 0 1 2 2 2
  spline S38 degree 2 poles (-33.4172, 87.7491) (-33.185, 87.8948) (-32.7083, 87.9936) (-32.3378, 87.9936) knots 0 0 0 1 2 2 2
  line L84 (-32.3378, 87.9936) -> (-31.6363, 87.9936)
  line L85 (-31.6363, 87.9936) -> (-31.6363, 84.9456)
  line L86 (-31.6363, 84.9456) -> (-32.3304, 84.9456)
  spline S39 degree 2 poles (-32.3304, 84.9456) (-32.7602, 84.9456) (-33.2492, 85.0741) (-33.4221, 85.1877) knots 0 0 0 1 2 2 2
  spline S40 degree 2 poles (-33.4221, 85.1877) (-33.7161, 85.3828) (-34.0396, 86.0275) (-34.0396, 86.4721) knots 0 0 0 1 2 2 2
  spline S41 degree 2 poles (-33.6173, 86.4672) (-33.6173, 86.1164) (-33.3851, 85.62) (-33.1554, 85.4792) knots 0 0 0 1 2 2 2
  spline S42 degree 2 poles (-33.1554, 85.4792) (-32.9923, 85.3828) (-32.6243, 85.2964) (-32.3501, 85.2964) knots 0 0 0 1 2 2 2
  line L87 (-32.3501, 85.2964) -> (-32.0414, 85.2964)
  line L88 (-32.0414, 85.2964) -> (-32.0414, 87.6429)
  line L89 (-32.0414, 87.6429) -> (-32.3501, 87.6429)
  spline S43 degree 2 poles (-32.3501, 87.6429) (-32.6194, 87.6429) (-33.0269, 87.5565) (-33.1924, 87.4404) knots 0 0 0 1 2 2 2
  spline S44 degree 2 poles (-33.1924, 87.4404) (-33.4048, 87.2971) (-33.6173, 86.8229) (-33.6173, 86.4672) knots 0 0 0 1 2 2 2
  line L90 (-34.4793, 87.9936) -> (-34.4793, 84.9456)
  line L91 (-34.4793, 84.9456) -> (-36.3862, 84.9456)
  line L92 (-36.3862, 84.9456) -> (-36.3862, 85.3063)
  line L93 (-36.3862, 85.3063) -> (-34.8844, 85.3063)
  line L94 (-34.8844, 85.3063) -> (-34.8844, 86.1411)
  line L95 (-34.8844, 86.1411) -> (-36.2849, 86.1411)
  line L96 (-36.2849, 86.1411) -> (-36.2849, 86.5018)
  line L97 (-36.2849, 86.5018) -> (-34.8844, 86.5018)
  line L98 (-34.8844, 86.5018) -> (-34.8844, 87.633)
  line L99 (-34.8844, 87.633) -> (-36.3862, 87.633)
  line L100 (-36.3862, 87.633) -> (-36.3862, 87.9936)
  line L101 (-36.3862, 87.9936) -> (-34.4793, 87.9936)
  line L102 (-39.1896, 87.9936) -> (-38.6635, 87.9936)
  line L103 (-38.6635, 87.9936) -> (-37.7002, 86.7809)
  line L104 (-37.7002, 86.7809) -> (-37.2358, 86.7809)
  line L105 (-37.2358, 86.7809) -> (-37.2358, 87.9936)
  line L106 (-37.2358, 87.9936) -> (-36.8308, 87.9936)
  line L107 (-36.8308, 87.9936) -> (-36.8308, 84.9456)
  line L108 (-36.8308, 84.9456) -> (-37.6162, 84.9456)
  spline S45 degree 2 poles (-37.6162, 84.9456) (-37.878, 84.9456) (-38.2313, 85.0025) (-38.3918, 85.1062) knots 0 0 0 1 2 2 2
  spline S46 degree 2 poles (-38.3918, 85.1062) (-38.5524, 85.2099) (-38.7376, 85.5335) (-38.7376, 85.7731) knots 0 0 0 1 2 2 2
  spline S47 degree 2 poles (-38.7376, 85.7731) (-38.7376, 86.1066) (-38.3967, 86.5586) (-38.1053, 86.6672) knots 0 0 0 1 2 2 2
  line L109 (-38.1053, 86.6672) -> (-39.1896, 87.9936)
  spline S48 degree 2 poles (-38.3152, 85.8052) (-38.3152, 85.6718) (-38.2214, 85.4668) (-38.1226, 85.4001) knots 0 0 0 1 2 2 2
  spline S49 degree 2 poles (-38.1226, 85.4001) (-38.0361, 85.3433) (-37.8064, 85.2964) (-37.6384, 85.2964) knots 0 0 0 1 2 2 2
  line L110 (-37.6384, 85.2964) -> (-37.2358, 85.2964)
  line L111 (-37.2358, 85.2964) -> (-37.2358, 86.4425)
  line L112 (-37.2358, 86.4425) -> (-37.5915, 86.4425)
  spline S50 degree 2 poles (-37.5915, 86.4425) (-37.7669, 86.4425) (-38.046, 86.3807) (-38.1423, 86.2844) knots 0 0 0 1 2 2 2
  spline S51 degree 2 poles (-38.1423, 86.2844) (-38.2313, 86.2004) (-38.3152, 85.9633) (-38.3152, 85.8052) knots 0 0 0 1 2 2 2
  spline S52 degree 2 poles (-8.5268, 91.4881) (-8.5268, 92.3081) (-8.0501, 93.0763) (-7.5537, 93.0763) knots 0 0 0 1 2 2 2
  spline S53 degree 2 poles (-7.5537, 93.0763) (-7.0498, 93.0763) (-6.578, 92.2933) (-6.578, 91.4906) knots 0 0 0 1 2 2 2
  spline S54 degree 2 poles (-6.578, 91.4906) (-6.578, 90.6656) (-7.0547, 89.9023) (-7.5537, 89.9023) knots 0 0 0 1 2 2 2
  spline S55 degree 2 poles (-7.5537, 89.9023) (-8.0551, 89.9023) (-8.5268, 90.6928) (-8.5268, 91.4881) knots 0 0 0 1 2 2 2
  spline S56 degree 2 poles (-8.0032, 92.4168) (-8.0625, 92.2662) (-8.1119, 91.8018) (-8.1119, 91.4881) knots 0 0 0 1 2 2 2
  spline S57 degree 2 poles (-8.1119, 91.4881) (-8.1119, 91.1744) (-8.0625, 90.7125) (-8.0007, 90.5569) knots 0 0 0 1 2 2 2
  spline S58 degree 2 poles (-8.0007, 90.5569) (-7.939, 90.4013) (-7.7241, 90.2407) (-7.5537, 90.2407) knots 0 0 0 1 2 2 2
  spline S59 degree 2 poles (-7.5537, 90.2407) (-7.3832, 90.2407) (-7.1634, 90.4013) (-7.0992, 90.5618) knots 0 0 0 1 2 2 2
  spline S60 degree 2 poles (-7.0992, 90.5618) (-7.0374, 90.7175) (-6.993, 91.1917) (-6.993, 91.4906) knots 0 0 0 1 2 2 2
  spline S61 degree 2 poles (-6.993, 91.4906) (-6.993, 91.8117) (-7.0325, 92.2415) (-7.0967, 92.4094) knots 0 0 0 1 2 2 2
  spline S62 degree 2 poles (-7.0967, 92.4094) (-7.156, 92.5675) (-7.3758, 92.7379) (-7.5537, 92.7379) knots 0 0 0 1 2 2 2
  spline S63 degree 2 poles (-7.5537, 92.7379) (-7.7216, 92.7379) (-7.9414, 92.5774) (-8.0032, 92.4168) knots 0 0 0 1 2 2 2
  line L113 (-10.8314, 90.4211) -> (-9.5124, 93.0121)
  line L114 (-9.5124, 93.0121) -> (-9.0777, 93.0121)
  line L115 (-9.0777, 93.0121) -> (-10.4707, 90.3222)
  line L116 (-10.4707, 90.3222) -> (-8.8973, 90.3222)
  line L117 (-8.8973, 90.3222) -> (-8.8973, 89.9641)
  line L118 (-8.8973, 89.9641) -> (-10.8314, 89.9641)
  line L119 (-10.8314, 89.9641) -> (-10.8314, 90.4211)
  line L120 (-11.8589, 93.0121) -> (-11.3698, 93.0121)
  line L121 (-11.3698, 93.0121) -> (-11.3698, 92.4292)
  line L122 (-11.3698, 92.4292) -> (-11.8589, 92.4292)
  line L123 (-11.8589, 92.4292) -> (-11.8589, 93.0121)
  line L124 (-14.2005, 93.0121) -> (-12.7135, 93.0121)
  line L125 (-12.7135, 93.0121) -> (-12.7135, 92.7009)
  line L126 (-12.7135, 92.7009) -> (-13.2668, 92.7009)
  line L127 (-13.2668, 92.7009) -> (-13.2668, 90.6582)
  line L128 (-13.2668, 90.6582) -> (-12.7135, 90.6582)
  line L129 (-12.7135, 90.6582) -> (-12.7135, 90.3791)
  spline S64 degree 2 poles (-12.7135, 90.3791) (-13.0272, 90.3791) (-13.3236, 90.2012) (-13.3434, 89.9542) knots 0 0 0 1 2 2 2
  line L130 (-13.3434, 89.9542) -> (-13.6595, 89.9542)
  line L131 (-13.6595, 89.9542) -> (-13.6595, 92.7009)
  line L132 (-13.6595, 92.7009) -> (-14.2005, 92.7009)
  line L133 (-14.2005, 92.7009) -> (-14.2005, 93.0121)
  spline S65 degree 2 poles (-16.6878, 92.0241) (-16.6878, 92.2587) (-16.5322, 92.6564) (-16.4013, 92.7898) knots 0 0 0 1 2 2 2
  spline S66 degree 2 poles (-16.4013, 92.7898) (-16.2654, 92.9306) (-15.9245, 93.0763) (-15.7195, 93.0763) knots 0 0 0 1 2 2 2
  spline S67 degree 2 poles (-15.7195, 93.0763) (-15.5145, 93.0763) (-15.1761, 92.938) (-15.0477, 92.7997) knots 0 0 0 1 2 2 2
  spline S68 degree 2 poles (-15.0477, 92.7997) (-14.8896, 92.6342) (-14.7118, 92.0784) (-14.7118, 91.6733) knots 0 0 0 1 2 2 2
  spline S69 degree 2 poles (-14.7118, 91.6733) (-14.7118, 91.2757) (-14.8748, 90.6359) (-15.0452, 90.3988) knots 0 0 0 1 2 2 2
  spline S70 degree 2 poles (-15.0452, 90.3988) (-15.2107, 90.1666) (-15.7343, 89.9073) (-16.0777, 89.9073) knots 0 0 0 1 2 2 2
  spline S71 degree 2 poles (-16.0777, 89.9073) (-16.1789, 89.9073) (-16.3568, 89.927) (-16.4235, 89.9493) knots 0 0 0 1 2 2 2
  line L134 (-16.4235, 89.9493) -> (-16.4235, 90.342)
  line L135 (-16.4235, 90.342) -> (-16.4062, 90.342)
  spline S72 degree 2 poles (-16.4062, 90.342) (-16.3494, 90.3124) (-16.1419, 90.2605) (-16.0233, 90.2605) knots 0 0 0 1 2 2 2
  spline S73 degree 2 poles (-16.0233, 90.2605) (-15.643, 90.2605) (-15.1761, 90.7743) (-15.1317, 91.2781) knots 0 0 0 1 2 2 2
  spline S74 degree 2 poles (-15.1317, 91.2781) (-15.2774, 91.1769) (-15.5837, 91.0657) (-15.7665, 91.0657) knots 0 0 0 1 2 2 2
  spline S75 degree 2 poles (-15.7665, 91.0657) (-15.9443, 91.0657) (-16.2111, 91.1374) (-16.3568, 91.246) knots 0 0 0 1 2 2 2
  spline S76 degree 2 poles (-16.3568, 91.246) (-16.5248, 91.372) (-16.6878, 91.7623) (-16.6878, 92.0241) knots 0 0 0 1 2 2 2
  spline S77 degree 2 poles (-16.2728, 92.0414) (-16.2728, 91.8537) (-16.174, 91.5992) (-16.0653, 91.5103) knots 0 0 0 1 2 2 2
  spline S78 degree 2 poles (-16.0653, 91.5103) (-15.9838, 91.4461) (-15.7813, 91.4041) (-15.6751, 91.4041) knots 0 0 0 1 2 2 2
  spline S79 degree 2 poles (-15.6751, 91.4041) (-15.5318, 91.4041) (-15.2626, 91.4906) (-15.1317, 91.5721) knots 0 0 0 1 2 2 2
  spline S80 degree 2 poles (-15.1317, 91.5721) (-15.1292, 91.6165) (-15.1243, 91.7005) (-15.1243, 91.7647) knots 0 0 0 1 2 2 2
  spline S81 degree 2 poles (-15.1243, 91.7647) (-15.1243, 92.0809) (-15.2478, 92.4687) (-15.3416, 92.57) knots 0 0 0 1 2 2 2
  spline S82 degree 2 poles (-15.3416, 92.57) (-15.4281, 92.6663) (-15.6158, 92.7429) (-15.722, 92.7429) knots 0 0 0 1 2 2 2
  spline S83 degree 2 poles (-15.722, 92.7429) (-15.969, 92.7429) (-16.2728, 92.3921) (-16.2728, 92.0414) knots 0 0 0 1 2 2 2
  line L136 (-17.7029, 93.0121) -> (-17.2139, 93.0121)
  line L137 (-17.2139, 93.0121) -> (-17.2139, 92.4292)
  line L138 (-17.2139, 92.4292) -> (-17.7029, 92.4292)
  line L139 (-17.7029, 92.4292) -> (-17.7029, 93.0121)
  line L140 (-20.1977, 93.0121) -> (-18.318, 93.0121)
  line L141 (-18.318, 93.0121) -> (-18.318, 92.5798)
  spline S84 degree 2 poles (-18.318, 92.5798) (-18.5205, 92.3897) (-18.8811, 92.0364) (-19.054, 91.8463) knots 0 0 0 1 2 2 2
  spline S85 degree 2 poles (-19.054, 91.8463) (-19.4023, 91.4634) (-19.6567, 91.004) (-19.6567, 90.7594) knots 0 0 0 1 2 2 2
  spline S86 degree 2 poles (-19.6567, 90.7594) (-19.6567, 90.631) (-19.5777, 90.4383) (-19.5061, 90.3766) knots 0 0 0 1 2 2 2
  spline S87 degree 2 poles (-19.5061, 90.3766) (-19.4344, 90.3148) (-19.2467, 90.2531) (-19.1331, 90.2531) knots 0 0 0 1 2 2 2
  spline S88 degree 2 poles (-19.1331, 90.2531) (-19.0244, 90.2531) (-18.8021, 90.3074) (-18.7008, 90.3494) knots 0 0 0 1 2 2 2
  spline S89 degree 2 poles (-18.7008, 90.3494) (-18.6144, 90.384) (-18.4538, 90.4828) (-18.4044, 90.5174) knots 0 0 0 1 2 2 2
  line L142 (-18.4044, 90.5174) -> (-18.3822, 90.5174)
  line L143 (-18.3822, 90.5174) -> (-18.3822, 90.0827)
  spline S90 degree 2 poles (-18.3822, 90.0827) (-18.5082, 90.0209) (-18.9602, 89.8999) (-19.1627, 89.8999) knots 0 0 0 1 2 2 2
  spline S91 degree 2 poles (-19.1627, 89.8999) (-19.59, 89.8999) (-20.0717, 90.3519) (-20.0717, 90.7372) knots 0 0 0 1 2 2 2
  spline S92 degree 2 poles (-20.0717, 90.7372) (-20.0717, 90.9175) (-19.9877, 91.2189) (-19.9136, 91.3473) knots 0 0 0 1 2 2 2
  spline S93 degree 2 poles (-19.9136, 91.3473) (-19.8395, 91.4807) (-19.6246, 91.7425) (-19.5061, 91.8685) knots 0 0 0 1 2 2 2
  spline S94 degree 2 poles (-19.5061, 91.8685) (-19.3134, 92.0784) (-18.8416, 92.528) (-18.7008, 92.6589) knots 0 0 0 1 2 2 2
  line L144 (-18.7008, 92.6589) -> (-20.1977, 92.6589)